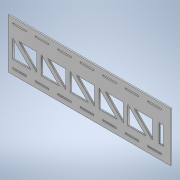
# Autodesk Inventor part: Bridge2
Saved by Autodesk Inventor 2022 (Build 260153000, 153)
## iProperties
Created: 2022-02-25
Part Number: Bridge2
Material: Generic
Document SubType Name: Modeling
Designer: anjarwala7025
Density: 1 g/cm^3
Appearance: Default
Author: anjarwala7025
Autodesk Inventor part; units mm, degrees
ref_plane "YZ Plane" through (0, 0, 0) normal (1, 0, 0) x (0, 1, 0)
ref_plane "XZ Plane" through (0, 0, 0) normal (0, 1, 0) x (-1, 0, 0)
ref_plane "XY Plane" through (0, 0, 0) normal (0, 0, 1) x (1, 0, 0)
sketch "Sketch1" plane through (0, 0, 0) normal (0, 0, 1) x (1, 0, 0)
  line L0 (0, 0) -> (457.2, 0)
  line L1 (457.2, 0) -> (457.2, 139.7)
  line L2 (457.2, 139.7) -> (0, 139.7)
  line L3 (0, 139.7) -> (0, 0)
  dimension "d0" = 457.2
  dimension "d1" = 139.7
  constraints: 8 end point, 2 parallel, 1 horizontal, 1 perpendicular
  measures "d0" distance of L1.end L2.end
  measures "d1" distance of L0.end L1.end
extrude "Extrusion1" add sketch "Sketch1" along normal blind 3.175
sketch "Sketch2" plane through (0, 0, 3.175) normal (0, 0, 1) x (1, 0, 0)
  line L0 (0, 139.7) -> (0, 0) projected
  line L1 (0, 114.3) -> (457.2, 114.3)
  line L2 (457.2, 139.7) -> (0, 139.7) projected
  line L3 (0, 38.1) -> (457.2, 38.1)
  line L4 (457.2, 0) -> (457.2, 139.7) projected
  line L5 (0, 0) -> (457.2, 0) projected
  line L6 (12.7, 17.6917) -> (50.8, 17.6917)
  line L7 (50.8, 17.6917) -> (50.8, 14.5167)
  line L8 (50.8, 14.5167) -> (12.7, 14.5167)
  line L9 (12.7, 14.5167) -> (12.7, 17.6917)
  line L10 (12.7, 127) -> (50.8, 127)
  line L11 (50.8, 127) -> (50.8, 123.825)
  line L12 (50.8, 123.825) -> (12.7, 123.825)
  line L13 (12.7, 123.825) -> (12.7, 127)
  line L14 (76.2, 127) -> (114.3, 127)
  line L15 (114.3, 127) -> (114.3, 123.825)
  line L16 (114.3, 123.825) -> (76.2, 123.825)
  line L17 (76.2, 123.825) -> (76.2, 127)
  line L18 (139.7, 127) -> (177.8, 127)
  line L19 (177.8, 127) -> (177.8, 123.825)
  line L20 (177.8, 123.825) -> (139.7, 123.825)
  line L21 (139.7, 123.825) -> (139.7, 127)
  line L22 (203.2, 127) -> (241.3, 127)
  line L23 (241.3, 127) -> (241.3, 123.825)
  line L24 (241.3, 123.825) -> (203.2, 123.825)
  line L25 (203.2, 123.825) -> (203.2, 127)
  line L26 (266.7, 127) -> (304.8, 127)
  line L27 (304.8, 127) -> (304.8, 123.825)
  line L28 (304.8, 123.825) -> (266.7, 123.825)
  line L29 (266.7, 123.825) -> (266.7, 127)
  line L30 (330.2, 127) -> (368.3, 127)
  line L31 (368.3, 127) -> (368.3, 123.825)
  line L32 (368.3, 123.825) -> (330.2, 123.825)
  line L33 (330.2, 123.825) -> (330.2, 127)
  line L34 (393.7, 127) -> (431.8, 127)
  line L35 (431.8, 127) -> (431.8, 123.825)
  line L36 (431.8, 123.825) -> (393.7, 123.825)
  line L37 (393.7, 123.825) -> (393.7, 127)
  line L38 (76.2, 17.6917) -> (114.3, 17.6917)
  line L39 (114.3, 17.6917) -> (114.3, 14.5167)
  line L40 (114.3, 14.5167) -> (76.2, 14.5167)
  line L41 (76.2, 14.5167) -> (76.2, 17.6917)
  line L42 (139.7, 17.6917) -> (177.8, 17.6917)
  line L43 (177.8, 17.6917) -> (177.8, 14.5167)
  line L44 (177.8, 14.5167) -> (139.7, 14.5167)
  line L45 (139.7, 14.5167) -> (139.7, 17.6917)
  line L46 (203.2, 17.6917) -> (241.3, 17.6917)
  line L47 (241.3, 17.6917) -> (241.3, 14.5167)
  line L48 (241.3, 14.5167) -> (203.2, 14.5167)
  line L49 (203.2, 14.5167) -> (203.2, 17.6917)
  line L50 (266.7, 17.6917) -> (304.8, 17.6917)
  line L51 (304.8, 17.6917) -> (304.8, 14.5167)
  line L52 (304.8, 14.5167) -> (266.7, 14.5167)
  line L53 (266.7, 14.5167) -> (266.7, 17.6917)
  line L54 (330.2, 17.6917) -> (368.3, 17.6917)
  line L55 (368.3, 17.6917) -> (368.3, 14.5167)
  line L56 (368.3, 14.5167) -> (330.2, 14.5167)
  line L57 (330.2, 14.5167) -> (330.2, 17.6917)
  line L58 (393.7, 17.6917) -> (431.8, 17.6917)
  line L59 (431.8, 17.6917) -> (431.8, 14.5167)
  line L60 (431.8, 14.5167) -> (393.7, 14.5167)
  line L61 (393.7, 14.5167) -> (393.7, 17.6917)
  dimension "d106" = 3.175
  dimension "d107" = 25.4
  dimension "d108" = 25.4
  dimension "d109" = 12.7
  dimension "d110" = 12.7
  dimension "d111" = 25.4
  dimension "d112" = 12.7
  dimension "d113" = 25.4
  dimension "d114" = 12.7
  dimension "d115" = 25.4
  dimension "d116" = 12.7
  dimension "d117" = 25.4
  dimension "d118" = 12.7
  dimension "d119" = 25.4
  dimension "d120" = 12.7
  dimension "d121" = 12.7
  dimension "d122" = 38.1
  dimension "d123" = 38.1
  dimension "d124" = 38.1
  dimension "d125" = 38.1
  dimension "d126" = 38.1
  dimension "d127" = 38.1
  dimension "d128" = 3.175
  dimension "d129" = 3.175
  dimension "d130" = 3.175
  dimension "d131" = 3.175
  dimension "d132" = 3.175
  dimension "d133" = 3.175
  dimension "d134" = 25.4
  dimension "d135" = 38.1
  dimension "d136" = 25.4
  dimension "d137" = 38.1
  dimension "d138" = 25.4
  dimension "d139" = 38.1
  dimension "d140" = 25.4
  dimension "d141" = 38.1
  dimension "d142" = 25.4
  dimension "d143" = 38.1
  dimension "d144" = 25.4
  dimension "d145" = 38.1
  dimension "d146" = 25.4
  dimension "d147" = 38.1
  dimension "d148" = 14.5167
  dimension "d150" = 14.5167
  dimension "d151" = 3.175
  dimension "d152" = 3.175
  constraints: 116 end point, 29 parallel, 15 horizontal, 14 perpendicular, 13 point on line
  measures "d106" distance between parallel lines of L36 L34
  measures "d107" distance between parallel lines of L4 L35
  measures "d108" distance between parallel lines of L31 L37
  measures "d109" distance between parallel lines of L2 L34
  measures "d110" distance between parallel lines of L2 L30
  measures "d111" distance between parallel lines of L27 L33
  measures "d112" distance between parallel lines of L2 L26
  measures "d113" distance between parallel lines of L23 L29
  measures "d114" distance between parallel lines of L2 L22
  measures "d115" distance between parallel lines of L19 L25
  measures "d116" distance between parallel lines of L2 L18
  measures "d117" distance between parallel lines of L15 L21
  measures "d118" distance between parallel lines of L2 L14
  measures "d119" distance between parallel lines of L11 L17
  measures "d120" distance between parallel lines of L2 L10
  measures "d121" distance between parallel lines of L0 L13
  measures "d122" distance between parallel lines of L37 L35
  measures "d123" distance between parallel lines of L33 L31
  measures "d124" distance between parallel lines of L29 L27
  measures "d125" distance between parallel lines of L25 L23
  measures "d126" distance between parallel lines of L21 L19
  measures "d127" distance between parallel lines of L17 L15
  measures "d128" distance between parallel lines of L32 L30
  measures "d129" distance between parallel lines of L28 L26
  measures "d130" distance between parallel lines of L24 L22
  measures "d131" distance between parallel lines of L20 L18
  measures "d132" distance between parallel lines of L16 L14
  measures "d133" distance between parallel lines of L12 L10
  measures "d134" distance between parallel lines of L4 L59
  measures "d135" distance between parallel lines of L61 L59
  measures "d136" distance between parallel lines of L55 L61
  measures "d137" distance between parallel lines of L57 L55
  measures "d138" distance between parallel lines of L51 L57
  measures "d139" distance between parallel lines of L53 L51
  measures "d140" distance between parallel lines of L47 L53
  measures "d141" distance between parallel lines of L49 L47
  measures "d142" distance between parallel lines of L43 L49
  measures "d143" distance between parallel lines of L45 L43
  measures "d144" distance between parallel lines of L39 L45
  measures "d145" distance between parallel lines of L41 L39
  measures "d146" distance between parallel lines of L7 L41
  measures "d147" distance between parallel lines of L9 L7
  measures "d148" distance between parallel lines of L5 L8
  measures "d150" distance between parallel lines of L5 L60
  measures "d151" distance between parallel lines of L60 L58
  measures "d152" distance between parallel lines of L8 L6
extrude "Extrusion2" cut sketch "Sketch2" against normal through all contours L6 L7 L8 L9 | L10 L11 L12 L13 | L14 L15 L16 L17 | L18 L19 L20 L21 | L22 L23 L24 L25 | L26 L27 L28 L29 | L30 L31 L32 L33 | L34 L35 L36 L37 | L38 L39 L40 L41 | L42 L43 L44 L45 | L46 L47 L48 L49 | L50 L51 L52 L53 | L54 L55 L56 L57 | L58 L59 L60 L61
sketch "Sketch3" plane through (0, 0, 3.175) normal (0, 0, 1) x (1, 0, 0)
  line L0 (0, 139.7) -> (0, 0) projected
  line L1 (0, 38.1) -> (457.2, 38.1)
  line L2 (457.2, 0) -> (457.2, 139.7) projected
  line L3 (0, 0) -> (457.2, 0) projected
  line L4 (0, 101.6) -> (457.2, 101.6)
  line L5 (457.2, 139.7) -> (0, 139.7) projected
  line L6 (12.7, 88.9) -> (12.7, 38.1)
  line L7 (12.7, 38.1) -> (63.5, 38.1)
  line L8 (63.5, 38.1) -> (12.7, 88.9)
  line L9 (29.5512, 90.0093) -> (80.3512, 39.2093)
  line L10 (80.3512, 39.2093) -> (80.3512, 90.0093)
  line L11 (80.3512, 90.0093) -> (29.5512, 90.0093)
  line L12 (93.0512, 38.1) -> (93.0512, 88.9)
  line L13 (93.0512, 38.1) -> (143.8512, 38.1)
  line L14 (143.8512, 38.1) -> (93.0512, 88.9)
  line L15 (111.0117, 88.9) -> (161.8117, 88.9)
  line L16 (161.8117, 88.9) -> (161.8117, 38.1)
  line L17 (161.8117, 38.1) -> (111.0117, 88.9)
  line L18 (174.5117, 88.9) -> (174.5117, 38.1)
  line L19 (174.5117, 38.1) -> (225.3117, 38.1)
  line L20 (225.3117, 38.1) -> (174.5117, 88.9)
  line L21 (243.2722, 38.1) -> (243.2722, 88.9)
  line L22 (243.2722, 88.9) -> (192.4722, 88.9)
  line L23 (192.4722, 88.9) -> (243.2722, 38.1)
  line L24 (255.9722, 88.9) -> (255.9722, 38.1)
  line L25 (255.9722, 38.1) -> (306.7722, 38.1)
  line L26 (306.7722, 38.1) -> (255.9722, 88.9)
  line L27 (273.9327, 88.9) -> (324.7327, 88.9)
  line L28 (324.7327, 88.9) -> (324.7327, 38.1)
  line L29 (324.7327, 38.1) -> (273.9327, 88.9)
  line L30 (337.4327, 88.9) -> (337.4327, 38.1)
  line L31 (337.4327, 38.1) -> (388.2327, 38.1)
  line L32 (388.2327, 38.1) -> (337.4327, 88.9)
  line L33 (355.3933, 88.9) -> (406.1933, 88.9)
  line L34 (406.1933, 88.9) -> (406.1933, 38.1)
  line L35 (406.1933, 38.1) -> (355.3933, 88.9)
  line L36 (425.2433, 88.9) -> (437.9433, 88.9)
  line L37 (437.9433, 88.9) -> (437.9433, 38.1)
  line L38 (437.9433, 38.1) -> (425.2433, 38.1)
  line L39 (425.2433, 38.1) -> (425.2433, 88.9)
  point P0 (355.3933, 88.9)
  dimension "d43" = 38.1
  dimension "d44" = 38.1
  dimension "d47" = 12.7
  dimension "d49" = 50.8
  dimension "d52" = 12.7
  dimension "d55" = 50.8
  dimension "d62" = 50.8
  dimension "d64" = 12.7
  dimension "d65" = 12.7
  dimension "d66" = 50.8
  dimension "d67" = 50.8
  dimension "d68" = 12.7
  dimension "d69" = 12.7
  dimension "d71" = 50.8
  dimension "d72" = 50.8
  dimension "d73" = 12.7
  dimension "d74" = 12.7
  dimension "d75" = 50.8
  dimension "d76" = 12.7
  dimension "d77" = 12.7
  dimension "d78" = 50.8
  dimension "d79" = 50.8
  dimension "d80" = 12.7
  dimension "d81" = 12.7
  dimension "d82" = 50.8
  dimension "d83" = 50.8
  dimension "d84" = 12.7
  dimension "d85" = 12.7
  dimension "d86" = 50.8
  dimension "d87" = 50.8
  dimension "d89" = 12.7
  dimension "d90" = 12.7
  dimension "d91" = 12.7
  dimension "d92" = 50.8
  dimension "d93" = 50.8
  dimension "d94" = 50.8
  dimension "d96" = 19.05
  dimension "d153" = 0
  dimension "d154" = 0
  constraints: 72 end point, 13 perpendicular, 6 vertical, 5 horizontal, 4 point on line, 3 parallel
  measures "d43" distance between parallel lines of L3 L1
  measures "d44" distance between parallel lines of L4 L5
  measures "d47" distance between parallel lines of L6 L0
  measures "d49" distance of L10.end L9.start
  measures "d52" distance between parallel lines of L12 L10
  measures "d55" distance of L15.start L15.end
  measures "d62" distance of L12.start L13.end
  measures "d64" distance between parallel lines of L9 L8
  measures "d65" distance between parallel lines of L17 L14
  measures "d66" distance of L6.start L6.end
  measures "d67" distance of L18.end L19.end
  measures "d68" distance between parallel lines of L18 L16
  measures "d69" distance from line of L4 L18.start
  measures "d71" distance of L21.start L21.end
  measures "d72" distance of L21.end L22.end
  measures "d73" distance between parallel lines of L23 L20
  measures "d74" distance between parallel lines of L4 L22
  measures "d75" distance of L24.end L25.end
  measures "d76" distance between parallel lines of L24 L21
  measures "d77" distance from line of L4 L24.start
  measures "d78" distance of L27.start L27.end
  measures "d79" distance of L27.end L28.end
  measures "d80" distance between parallel lines of L29 L26
  measures "d81" distance between parallel lines of L4 L27
  measures "d82" distance of L30.start L30.end
  measures "d83" distance of L30.end L31.end
  measures "d84" distance between parallel lines of L30 L28
  measures "d85" distance from line of L4 L30.start
  measures "d86" distance of L33.start L33.end
  measures "d87" distance of L33.end L34.end
  measures "d89" distance between parallel lines of L4 L33
  measures "d90" distance between parallel lines of L35 L32
  measures "d91" distance of L37.end L38.end
  measures "d92" distance of L6.end L7.end
  measures "d93" distance of L12.start L12.end
  measures "d94" distance of L24.start L24.end
  measures "d96" distance between parallel lines of L39 L34
  measures "d153" distance from line of L1 L7.end
  measures "d154" distance from line of L1 L13.end
extrude "Extrusion3" cut sketch "Sketch3" against normal through all contours L17 L15 L16 | L23 L22 L21 | L29 L27 L28 | L35 L33 L34 | L6 L8 L1 | L1 L39 L36 L37 | L12 L14 L1 | L1 L30 L32 | L18 L20 L1 | L1 L24 L26 | L11 L10 L9
body "Solid1"
